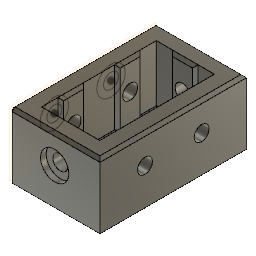
1-Display_Support_Endcaps_short_one (Autodesk Fusion 360 design; units mm, degrees)
Autodesk Fusion 360 part; units mm, degrees
sketch "Main Profile" plane through (0, 0, 0) normal (0, 0, 1) x (1, 0, 0)
  line L0 (10.25, -20.25) -> (-10.25, -20.25)
  line L1 (-10.25, -20.25) -> (-10.25, 20.25)
  line L2 (-10.25, 20.25) -> (10.25, 20.25)
  line L3 (10.25, 20.25) -> (10.25, -20.25)
  line L4 (10.25, -20.25) -> (-10.25, 20.25) construction
  line L5 (-10.25, -20.25) -> (10.25, 20.25) construction
  line L6 (-16, -25.9) -> (16, -25.9)
  line L7 (16, -25.9) -> (16, 25.9)
  line L8 (16, 25.9) -> (-16, 25.9)
  line L9 (-16, 25.9) -> (-16, -25.9)
  line L10 (-16, -25.9) -> (16, 25.9) construction
  line L11 (16, -25.9) -> (-16, 25.9) construction
  line L12 (-3.5, 19.25) -> (3.5, 19.25)
  line L13 (3.5, 19.25) -> (4.5, 20.25)
  line L14 (-3.5, 19.25) -> (-4.5, 20.25)
  line L15 (0, 20.25) -> (0, 19.25) construction
  line L16 (-9.25, 6.5) -> (-9.25, 13.5)
  line L17 (-9.25, 13.5) -> (-10.25, 14.5)
  line L18 (-9.25, 6.5) -> (-10.25, 5.5)
  line L19 (9.25, 13.5) -> (9.25, 6.5)
  line L20 (9.25, 6.5) -> (10.25, 5.5)
  line L21 (9.25, 13.5) -> (10.25, 14.5)
  line L22 (9.25, -13.5) -> (10.25, -14.5)
  line L23 (9.25, -6.5) -> (9.25, -13.5)
  line L24 (9.25, -6.5) -> (10.25, -5.5)
  line L25 (3.5, -19.25) -> (4.5, -20.25)
  line L26 (3.5, -19.25) -> (-3.5, -19.25)
  line L27 (-3.5, -19.25) -> (-4.5, -20.25)
  line L28 (-9.25, -13.5) -> (-10.25, -14.5)
  line L29 (-9.25, -13.5) -> (-9.25, -6.5)
  line L30 (-9.25, -6.5) -> (-10.25, -5.5)
  point P0 (0, 10)
  dimension "d1" = 40.5
  dimension "d2" = 20.5
  dimension "d3" = 32
  dimension "d4" = 51.8
  dimension "d5" = 1
  dimension "d6" = 135
  dimension "d7" = 7
  dimension "d8" = 135
  dimension "d9" = 10.25
  dimension "d11" = 360
  dimension "d13" = 360
  constraint perpendicular L0 L1
  constraint parallel L0 L2
  constraint parallel L1 L3
  constraint horizontal L0
  constraint coincident L4 origin
  constraint coincident L5 origin
  constraint perpendicular L6 L7
  constraint parallel L6 L8
  constraint parallel L7 L9
  constraint horizontal L6
  constraint coincident L10 origin
  constraint coincident L11 origin
  constraint horizontal L12
  constraint coincident L2 L13.end
  constraint coincident L2 L14.end
  constraint midpoint L2 L15.start
  constraint midpoint L12 L15.end
  constraint vertical L15
  constraint coincident L15 P0
  measures "d1" distance of L0.end L1.end
  measures "d2" distance of L1.end L2.end
  measures "d3" distance of L7.end L8.end
  measures "d4" distance of L6.end L7.end
  measures "d5" distance of L2 L12
  measures "d6" angle of L12 L14
  measures "d7" distance of L12.start L12.end
  measures "d8" angle of L12 L13
  measures "d9" distance of L15.start P0
extrude "Extrude1" add sketch "Main Profile" along normal blind 3 contours L0 L1 L2 L3 L12 L13 L14 L16 L17 L18 L19 L20 L21 L22 L23 L24 L25 L26 L27 L28 L29 L30 | L0 L25 L26 L27 | L3 L22 L23 L24 | L3 L19 L20 L21 | L1 L28 L29 L30 | L1 L16 L17 L18 | L2 L12 L13 L14 | L6 L7 L8 L9
extrude "Extrude2" add sketch "Main Profile" along normal blind 22.9 contours L0 L25 L26 L27 | L3 L22 L23 L24 | L3 L19 L20 L21 | L1 L28 L29 L30 | L1 L16 L17 L18 | L2 L12 L13 L14 | L6 L7 L8 L9
sketch "Short Side" plane through (0, 25.9, 0) normal (0, 1, 0) x (-1, 0, 0)
  line L0 (-16, 0) -> (16, 0)
  line L1 (16, 0) -> (16, 22.9)
  line L2 (16, 22.9) -> (-16, 22.9)
  line L3 (-16, 22.9) -> (-16, 0)
  circle A0 centre (0, 12.9) radius 5
  circle A1 centre (0, 12.9) radius 2.625
  dimension "d18" = 10
  dimension "d19" = 5.25
  dimension "d20" = 12.9
  constraint concentric A0 A1
  constraint vertical origin A0.centre
  measures "d18" diameter of A0
  measures "d19" diameter of A1
  measures "d20" distance of A0.centre origin
extrude "Extrude3" cut sketch "Short Side" against normal blind 63.819 contours A1
extrude "Extrude4" cut sketch "Short Side" against normal blind 2 contours A0
extrude "Extrude5" cut sketch "Short Side" along normal blind 2 from surface at -51.8 contours A0
sketch "Long Side" plane through (-16, 0, 0) normal (-1, 0, 0) x (0, -1, 0)
  line L0 (-25.9, 0) -> (25.9, 0)
  line L1 (25.9, 0) -> (25.9, 22.9)
  line L2 (25.9, 22.9) -> (-25.9, 22.9)
  line L3 (-25.9, 22.9) -> (-25.9, 0)
  circle A0 centre (-10, 12.9) radius 5
  circle A1 centre (-10, 12.9) radius 2.625
  circle A2 centre (10, 12.9) radius 5
  circle A3 centre (10, 12.9) radius 2.625
  dimension "d28" = 10
  dimension "d29" = 5.25
  dimension "d30" = 10
  dimension "d31" = 12.9
  dimension "d34" = 20
  dimension "d35" = 0
  constraint concentric A0 A1
  measures "d28" diameter of A0
  measures "d29" diameter of A1
  measures "d30" horizontal distance of origin A0.centre
  measures "d31" vertical distance of origin A0.centre
extrude "Extrude6" cut sketch "Long Side" against normal blind 62.946 contours A1 | A3
extrude "Extrude7" cut sketch "Long Side" against normal blind 2 contours A0 | A2
chamfer "Chamfer1" distance 1 angle 45 12 edges at (9.25, 10, 22.9) (9.25, -10, 22.9) (-9.25, -10, 22.9) (0, -19.25, 22.9) (-9.25, 10, 22.9) (0, 19.25, 22.9) (0, 25.9, 22.9) (16, 0, 22.9) (0, -25.9, 22.9) (-16, 0, 22.9) (-16, -25.9, 11.45) (-16, 25.9, 11.45)
named bodies: "1-Display_Support_Endcaps"
